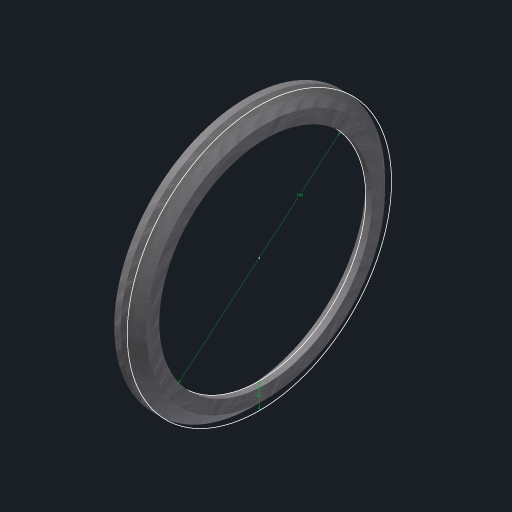
# Autodesk Inventor part: CIRCULO_fRONTAL
Saved by Autodesk Inventor 2024.3 (Build 283343000, 343)
## iProperties
Created: 2024-08-11
Part Number: CIRCULO_fRONTAL
Material: Steel, Mild, Welded
Document SubType Name: Modeling
Designer: Niler
Density: 7.85 g/cm^3
Appearance: Weld - Steel Mild
Author: Niler
Autodesk Inventor part; units mm, degrees
ref_plane "YZ Plane" through (0, 0, 0) normal (1, 0, 0) x (0, 1, 0)
ref_plane "XZ Plane" through (0, 0, 0) normal (0, 1, 0) x (-1, 0, 0)
ref_plane "XY Plane" through (0, 0, 0) normal (0, 0, 1) x (1, 0, 0)
sketch "Sketch1" plane through (0, 0, 0) normal (1, 0, 0) x (0, 1, 0)
  circle A0 centre (0, 0) radius 82.5
  circle A1 centre (0, 0) radius 102.5
  circle A2 centre (0, 0) radius 92.5
  dimension "d0" = 165
  dimension "d1" = 20
  dimension "d2" = 10
  constraints: 3 centre point, 1 coincident
  measures "d0" diameter of A0
  measures "d1" radial gap between concentric circles of A0 A1
  measures "d2" radial gap between concentric circles of A0 A2
extrude "Extrusion1" add sketch "Sketch1" along normal blind 5 contours A1 | A2
extrude "Extrusion2" add sketch "Sketch1" against normal blind 10 contours A1
chamfer "Chamfer1" distance 10 angle 45 1 edges at (5, -102.5, 0)
body "Solid1"
